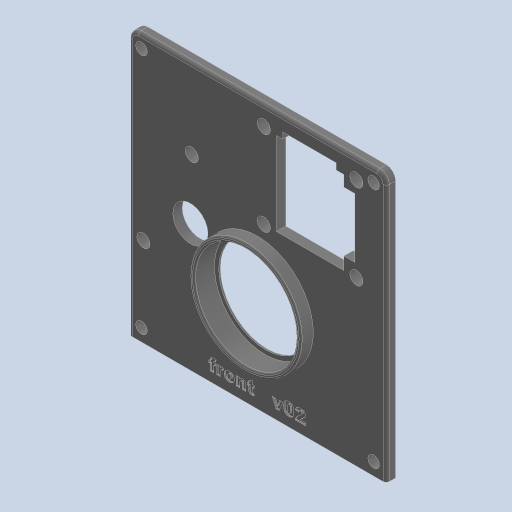
# Autodesk Inventor part: door_front_02
Saved by Autodesk Inventor 2024.4 (Build 284460030, 460C)
## iProperties
Created: 2026-07-13
Part Number: door_front_02
Material: Generic
Document SubType Name: Modeling
Designer: tooles01
Density: 1 g/cm^3
Appearance: Gray
d0: 3.000 mm
d1: 0.00 deg
d3: 32.500 mm
d4: 35.500 mm
d5: 7.000 mm
d6: 0.00 deg
d11: 29.750 mm
d12: 0.500 mm
d13: 0.00 deg
d14: 3.700 mm
d0_1: 36.000 mm
d3_1: 4.900 mm
d4_1: 3.000 mm
d5_1: 10.000 mm
d6_1: 2.000 mm
d7: 2.000 mm
d21: 30.000 mm
d22: 82.000 mm
d23: 4.000 mm
d24: 4.000 mm
d25: 4.000 mm
d26: 4.200 mm
d27: 35.000 mm
d28: 3.000 mm
d29: 4.900 mm
d32: 6.500 mm
d33: 2.000 mm
d34: 2.000 mm
d35: 10.000 mm
d37: 36.000 mm
d38: 2.000 mm
d39: 4.900 mm
d41: 4.200 mm
d48: 1.000 ul
d52: 0.00 deg
d53: 3.000 mm
d54: 34.500 mm
d55: 32.000 mm
d56: 3.000 mm
d57: 2.500 mm
d58: 27.000 mm
d59: 19.000 mm
d60: 7.000 mm
d61: 4.200 mm
d68: 55.000 mm
d69: 3.000 mm
d70: 1.000 mm
d71: 0.500 mm
d72: 40.000 mm
d73: 0.500 mm
d75: 5.000 mm
door_diameter: 36.000 mm
axle_width: 4.900 mm
axle_height: 3.200 mm
handle_height: 10.000 mm
spacing_height: 2.000 mm
spacing_width: 2.000 mm
door_diameter_1: 36.000 mm
handle_height_1: 10.000 mm
spacing_width_1: 2.000 mm
door_spacing_width_1: 2.000 mm
door_handle_height_1: 10.000 mm
door_door_diameter_1: 36.000 mm
door_axle_width_1: 4.900 mm
door_spacing_height_1: 2.000 mm
door_axle_width_2: 4.900 mm
door_axle_height_1: 3.200 mm
door_spacing_height_2: 2.000 mm
d76: 4.000 mm
d77: 9.200 mm
d78: 1.000 mm
d81: 1.000 mm
d83: 17.000 mm
d84: 2.000 mm
d85: 29.500 mm
d86: 6.000 mm
d88: 27.000 mm
d90: 4.000 mm
d91: 4.000 mm
d92: 4.000 mm
d93: 0.500 mm
d94: 1.500 mm
d98: 0.00 deg
d99: 4.000 mm
Author: tooles01
Autodesk Inventor part; units mm, degrees
ref_plane "YZ Plane" through (0, 0, 0) normal (1, 0, 0) x (0, 1, 0)
ref_plane "XZ Plane" through (0, 0, 0) normal (0, 1, 0) x (-1, 0, 0)
ref_plane "XY Plane" through (0, 0, 0) normal (0, 0, 1) x (1, 0, 0)
derived "door_02.ipt"
sketch "Sketch1: base" plane through (0, 0, 0) normal (0, 0, 1) x (1, 0, 0)
  line L0 (-41, 85) -> (41, 85)
  line L1 (41, 85) -> (41, 0)
  line L2 (41, 0) -> (-41, 0)
  line L3 (-41, 0) -> (-41, 85)
  circle A0 centre (0, 30) radius 16.25
  line L4 (-37, 81) -> (37, 81) construction
  line L5 (37, 81) -> (37, 4) construction
  line L6 (37, 4) -> (-37, 4) construction
  line L7 (-37, 4) -> (-37, 81) construction
  point P0 (0, 0)
  point P1 (0, 0)
  point P2 (0, 4)
  dimension "d3" = 32.5
  dimension "d21" = 30
  dimension "d22" = 82
  dimension "d23" = 4
  dimension "d24" = 4
  dimension "d25" = 4
  dimension "d68" = 55
  constraints: 16 end point, 6 perpendicular, 5 coincident, 2 horizontal, 2 midpoint, 2 vertical alignment, 1 centre point
  measures "d3" diameter of A0
  measures "d21" distance from line of L2 A0.centre
  measures "d22" distance of L1.end L2.end
  measures "d23" distance between parallel lines of L2 L6
  measures "d24" distance between parallel lines of L3 L7
  measures "d25" distance between parallel lines of L0 L4
  measures "d68" distance from line of L0 A0.centre
sketch "Sketch2: tube cover/stopper" plane through (0, 0, 0) normal (0, 0, 1) x (1, 0, 0)
  circle A0 centre (0, 30) radius 17.75
  circle A1 centre (0, 30) radius 14.875
  circle A2 centre (0, 30) radius 16.25 projected
  point P0 (0, 0)
  dimension "d4" = 35.5
  dimension "d11" = 29.75
  constraints: 3 coincident, 2 centre point
  measures "d4" diameter of A0
  measures "d11" diameter of A1
sketch "Sketch3: motor & door footprint" plane through (0, 0, 0) normal (0, 0, 1) x (1, 0, 0)
  circle A0 centre (-20.9777, 59.7729) radius 2.1 construction
  circle A1 centre (-36.3835, 28.3459) radius 2.1 construction
  line L0 (-20.9777, 59.7729) -> (-36.3835, 28.3459) construction
  line L1 (-18.8924, 41.9897) -> (-21.0492, 37.5899)
  line L2 (-21.0492, 37.5899) -> (-23.9225, 38.9985)
  line L3 (-23.9225, 38.9985) -> (-21.7657, 43.3982)
  line L4 (-21.7657, 43.3982) -> (-18.8924, 41.9897)
  line L5 (-22.8441, 41.1983) -> (-28.6806, 44.0594) construction
  line L6 (-22.6812, 46.0744) -> (-26.5987, 38.0829)
  line L7 (-26.5987, 38.0829) -> (-17.6195, 33.6813)
  line L8 (-13.7021, 41.6728) -> (-22.6812, 46.0744)
  circle A2 centre (0, 30) radius 18
  line L9 (0, 30) -> (-24.64, 42.0787) construction
  circle A3 centre (0, 30) radius 16.25 construction
  circle A4 centre (-19.0235, 64.2159) radius 18 construction
  line L10 (-25.1952, 47.307) -> (-26.1951, 37.3571) construction
  line L11 (-26.1951, 37.3571) -> (-17.3397, 36.4672) construction
  line L12 (-17.3397, 36.4672) -> (-16.3398, 46.417) construction
  line L13 (-18.8098, 41.8411) -> (-23.6852, 42.331) construction
  line L14 (-23.6852, 42.331) -> (-24.0052, 39.1471) construction
  line L15 (-24.0052, 39.1471) -> (-19.1297, 38.6571) construction
  line L16 (-19.1297, 38.6571) -> (-18.8098, 41.8411) construction
  line L17 (-19.0235, 64.2159) -> (-21.7674, 36.9121) construction
  circle A5 centre (-21.4075, 40.4941) radius 2.45 construction
  point P0 (0, 0)
  point P1 (-19.9708, 39.7898)
  point P2 (-21.5675, 38.9021)
  point P3 (-22.4859, 38.2942)
  point P4 (-18.9698, 40.2491)
  dimension "d26" = 4.2
  dimension "d27" = 34.9999
  dimension "door_axle_height_1" = 3.2
  dimension "door_axle_width_1" = 4.9
  dimension "d32" = 6.5
  dimension "door_spacing_height_1" = 2
  dimension "door_spacing_width_1" = 2
  dimension "door_handle_height_1" = 10
  dimension "door_door_diameter_1" = 36
  dimension "door_spacing_height_2" = 2
  dimension "door_axle_width_2" = 4.9
  constraints: 36 end point, 8 midpoint, 8 perpendicular, 7 parallel, 6 point on circle, 5 centre point, 5 coincident, 4 equal length, 4 point on line, 2 equal radius, 1 collinear, 1 other
  measures "d26" diameter of A0
  measures "d27" distance of L0.start L0.end
  measures "door_axle_height_1" distance of L3.end L1.start
  measures "door_axle_width_1" distance of L1.start L1.end
  measures "d32" distance from line of A0.centre L3
  measures "door_spacing_height_1" distance between parallel lines of L6 L3
  measures "door_spacing_width_1" distance between parallel lines of L8 L4
  measures "door_handle_height_1" distance of L8.start L6.start
  measures "door_door_diameter_1" diameter of A2
  measures "door_spacing_height_2" distance between parallel lines of L11 L15
  measures "door_axle_width_2" diameter of A5
sketch "Sketch4: holes for motor mount" plane through (0, 0, 0) normal (0, 0, 1) x (1, 0, 0)
  circle A0 centre (-21.4075, 40.4941) radius 2.45 construction
  circle A1 centre (-21.4075, 40.4941) radius 5.6
  circle A2 centre (-21.4075, 40.4941) radius 4.6 construction
  point P0 (0, 0)
  point P1 (-20.9777, 59.7729)
  point P2 (-36.3835, 28.3459)
  dimension "d77" = 9.2
  dimension "d78" = 1
  constraints: 2 centre point, 2 coincident
  measures "d77" diameter of A2
  measures "d78" radial gap between concentric circles of A1 A2
sketch "Sketch6: text" plane through (0, 0, 0) normal (0, 0, 1) x (1, 0, 0)
  line L0 (-20, 7) -> (20, 7) construction
  line L1 (20, 7) -> (20, 3) construction
  line L2 (20, 3) -> (-20, 3) construction
  line L3 (-20, 3) -> (-20, 7) construction
  line L4 (-13.9634, 5.8989) -> (-13.4321, 5.8989)
  line L5 (-13.4321, 5.8989) -> (-13.4321, 5.0866)
  line L6 (-13.4321, 5.0866) -> (-13.9634, 5.0866)
  line L7 (-13.9634, 5.0866) -> (-13.9634, 3)
  line L8 (-13.9634, 3) -> (-15.076, 3)
  line L9 (-15.076, 3) -> (-15.076, 5.0866)
  line L10 (-15.076, 5.0866) -> (-15.4918, 5.0866)
  line L11 (-15.4918, 5.0866) -> (-15.4918, 5.8989)
  line L12 (-15.4918, 5.8989) -> (-15.076, 5.8989)
  line L13 (-15.076, 5.8989) -> (-15.076, 6.0298)
  spline S0 degree 2 poles (-15.076, 6.0298) (-15.076, 6.2069) (-14.999, 6.6343) (-14.7911, 6.9038) (-14.41, 7.0693) (-14.0443, 7.0693) knots 0 0 0 1 2 3 4 4 4
  spline S1 degree 2 poles (-14.0443, 7.0693) (-13.7517, 7.0693) (-13.1973, 7) knots 0 0 0 1 1 1
  line L14 (-13.1973, 7) -> (-13.3205, 6.3301)
  spline S2 degree 2 poles (-13.3205, 6.3301) (-13.5168, 6.3609) (-13.64, 6.3609) knots 0 0 0 1 1 1
  spline S3 degree 2 poles (-13.64, 6.3609) (-13.7902, 6.3609) (-13.9211, 6.2608) (-13.948, 6.153) knots 0 0 0 1 2 2 2
  spline S4 degree 2 poles (-13.948, 6.153) (-13.9634, 6.0914) (-13.9634, 5.8989) knots 0 0 0 1 1 1
  line L15 (-13.0125, 5.8989) -> (-11.9731, 5.8989)
  line L16 (-11.9731, 5.8989) -> (-11.9731, 5.4254)
  spline S5 degree 2 poles (-11.9731, 5.4254) (-11.8229, 5.7334) (-11.5034, 5.9644) (-11.2685, 5.9644) knots 0 0 0 1 2 2 2
  spline S6 degree 2 poles (-11.2685, 5.9644) (-11.0221, 5.9644) (-10.7295, 5.8104) knots 0 0 0 1 1 1
  line L17 (-10.7295, 5.8104) -> (-11.0722, 5.0212)
  spline S7 degree 2 poles (-11.0722, 5.0212) (-11.2685, 5.102) (-11.384, 5.102) knots 0 0 0 1 1 1
  spline S8 degree 2 poles (-11.384, 5.102) (-11.6035, 5.102) (-11.7228, 4.9211) knots 0 0 0 1 1 1
  spline S9 degree 2 poles (-11.7228, 4.9211) (-11.8961, 4.667) (-11.8961, 3.9702) knots 0 0 0 1 1 1
  line L18 (-11.8961, 3.9702) -> (-11.8961, 3)
  line L19 (-11.8961, 3) -> (-13.0125, 3)
  line L20 (-13.0125, 3) -> (-13.0125, 5.8989)
  spline S10 degree 2 poles (-10.6756, 4.4398) (-10.6756, 5.1059) (-9.7825, 5.9644) (-9.0202, 5.9644) knots 0 0 0 1 2 2 2
  spline S11 degree 2 poles (-9.0202, 5.9644) (-8.1501, 5.9644) (-7.7074, 5.4601) knots 0 0 0 1 1 1
  spline S12 degree 2 poles (-7.7074, 5.4601) (-7.3494, 5.052) (-7.3494, 4.4591) knots 0 0 0 1 1 1
  spline S13 degree 2 poles (-7.3494, 4.4591) (-7.3494, 3.7892) (-8.2348, 2.9346) (-9.0164, 2.9346) knots 0 0 0 1 2 2 2
  spline S14 degree 2 poles (-9.0164, 2.9346) (-9.717, 2.9346) (-10.1482, 3.2887) knots 0 0 0 1 1 1
  spline S15 degree 2 poles (-10.1482, 3.2887) (-10.6756, 3.7276) (-10.6756, 4.4398) knots 0 0 0 1 1 1
  spline S16 degree 2 poles (-9.563, 4.4437) (-9.563, 4.0549) (-9.2512, 3.6853) (-9.0125, 3.6853) knots 0 0 0 1 2 2 2
  spline S17 degree 2 poles (-9.0125, 3.6853) (-8.7738, 3.6853) (-8.4658, 4.051) (-8.4658, 4.4552) knots 0 0 0 1 2 2 2
  spline S18 degree 2 poles (-8.4658, 4.4552) (-8.4658, 4.8287) (-8.7777, 5.1983) (-9.0048, 5.1983) knots 0 0 0 1 2 2 2
  spline S19 degree 2 poles (-9.0048, 5.1983) (-9.2474, 5.1983) (-9.563, 4.8248) (-9.563, 4.4437) knots 0 0 0 1 2 2 2
  line L21 (-6.8104, 5.8989) -> (-5.7748, 5.8989)
  line L22 (-5.7748, 5.8989) -> (-5.7748, 5.4254)
  spline S20 degree 2 poles (-5.7748, 5.4254) (-5.5438, 5.718) (-5.0664, 5.9644) (-4.7276, 5.9644) knots 0 0 0 1 2 2 2
  spline S21 degree 2 poles (-4.7276, 5.9644) (-4.2656, 5.9644) (-3.7459, 5.4139) (-3.7459, 4.8441) knots 0 0 0 1 2 2 2
  line L23 (-3.7459, 4.8441) -> (-3.7459, 3)
  line L24 (-3.7459, 3) -> (-4.8624, 3)
  line L25 (-4.8624, 3) -> (-4.8624, 4.5938)
  spline S22 degree 2 poles (-4.8624, 4.5938) (-4.8624, 4.8672) (-5.0626, 5.0943) (-5.2474, 5.0943) knots 0 0 0 1 2 2 2
  spline S23 degree 2 poles (-5.2474, 5.0943) (-5.4475, 5.0943) (-5.6978, 4.7902) (-5.6978, 4.3936) knots 0 0 0 1 2 2 2
  line L26 (-5.6978, 4.3936) -> (-5.6978, 3)
  line L27 (-5.6978, 3) -> (-6.8104, 3)
  line L28 (-6.8104, 3) -> (-6.8104, 5.8989)
  line L29 (-1.7401, 7) -> (-1.7401, 5.8989)
  line L30 (-1.7401, 5.8989) -> (-1.128, 5.8989)
  line L31 (-1.128, 5.8989) -> (-1.128, 5.0866)
  line L32 (-1.128, 5.0866) -> (-1.7401, 5.0866)
  line L33 (-1.7401, 5.0866) -> (-1.7401, 4.0587)
  spline S24 degree 2 poles (-1.7401, 4.0587) (-1.7401, 3.8739) (-1.7055, 3.8123) knots 0 0 0 1 1 1
  spline S25 degree 2 poles (-1.7055, 3.8123) (-1.6516, 3.7199) (-1.513, 3.7199) knots 0 0 0 1 1 1
  spline S26 degree 2 poles (-1.513, 3.7199) (-1.3898, 3.7199) (-1.1704, 3.7892) knots 0 0 0 1 1 1
  line L34 (-1.1704, 3.7892) -> (-1.0895, 3.0231)
  spline S27 degree 2 poles (-1.0895, 3.0231) (-1.5014, 2.9346) (-1.8595, 2.9346) knots 0 0 0 1 1 1
  spline S28 degree 2 poles (-1.8595, 2.9346) (-2.2714, 2.9346) (-2.6641, 3.1463) (-2.8527, 3.5813) (-2.8527, 4.0664) knots 0 0 0 1 2 3 3 3
  line L35 (-2.8527, 4.0664) -> (-2.8527, 5.0866)
  line L36 (-2.8527, 5.0866) -> (-3.2608, 5.0866)
  line L37 (-3.2608, 5.0866) -> (-3.2608, 5.8989)
  line L38 (-3.2608, 5.8989) -> (-2.8527, 5.8989)
  line L39 (-2.8527, 5.8989) -> (-2.8527, 6.4302)
  line L40 (-2.8527, 6.4302) -> (-1.7401, 7)
  line L41 (4.666, 5.8989) -> (5.821, 5.8989)
  line L42 (5.821, 5.8989) -> (6.3869, 4.0626)
  line L43 (6.3869, 4.0626) -> (6.9682, 5.8989)
  line L44 (6.9682, 5.8989) -> (8.0885, 5.8989)
  line L45 (8.0885, 5.8989) -> (6.8566, 3)
  line L46 (6.8566, 3) -> (5.871, 3)
  line L47 (5.871, 3) -> (4.666, 5.8989)
  spline S29 degree 2 poles (8.3041, 5.0173) (8.3041, 6.1569) (9.1242, 7.0693) (9.9634, 7.0693) knots 0 0 0 1 2 2 2
  spline S30 degree 2 poles (9.9634, 7.0693) (10.3677, 7.0693) (10.8835, 6.8691) (11.2108, 6.5496) (11.3994, 6.1992) (11.4572, 5.9644) knots 0 0 0 1 2 3 4 4 4
  spline S31 degree 2 poles (11.4572, 5.9644) (11.5688, 5.5178) (11.5688, 5.0289) knots 0 0 0 1 1 1
  spline S32 degree 2 poles (11.5688, 5.0289) (11.5688, 3.9394) (10.8335, 2.9307) (9.9326, 2.9307) knots 0 0 0 1 2 2 2
  spline S33 degree 2 poles (9.9326, 2.9307) (9.4283, 2.9307) (8.8085, 3.2541) (8.6083, 3.5659) knots 0 0 0 1 2 2 2
  spline S34 degree 2 poles (8.6083, 3.5659) (8.4658, 3.7854) (8.3041, 4.5515) (8.3041, 5.0173) knots 0 0 0 1 2 2 2
  spline S35 degree 2 poles (9.4052, 5.0135) (9.4052, 4.2474) (9.6747, 3.6891) (9.9288, 3.6891) knots 0 0 0 1 2 2 2
  spline S36 degree 2 poles (9.9288, 3.6891) (10.0982, 3.6891) (10.3484, 3.9278) (10.4639, 4.4398) (10.4639, 4.9827) knots 0 0 0 1 2 3 3 3
  spline S37 degree 2 poles (10.4639, 4.9827) (10.4639, 5.7796) (10.1944, 6.3301) (9.9249, 6.3301) knots 0 0 0 1 2 2 2
  spline S38 degree 2 poles (9.9249, 6.3301) (9.6516, 6.3301) (9.4052, 5.7719) (9.4052, 5.0135) knots 0 0 0 1 2 2 2
  line L48 (15.2839, 3) -> (11.95, 3)
  spline S39 degree 2 poles (11.95, 3) (12.0077, 3.4928) (12.589, 4.3628) (13.3898, 4.9557) knots 0 0 0 1 2 2 2
  spline S40 degree 2 poles (13.3898, 4.9557) (13.8749, 5.3176) (14.1482, 5.6949) (14.1482, 5.8643) knots 0 0 0 1 2 2 2
  spline S41 degree 2 poles (14.1482, 5.8643) (14.1482, 6.0491) (13.8787, 6.307) (13.6747, 6.307) knots 0 0 0 1 2 2 2
  spline S42 degree 2 poles (13.6747, 6.307) (13.4591, 6.307) (13.1896, 6.0414) (13.1434, 5.7026) knots 0 0 0 1 2 2 2
  line L49 (13.1434, 5.7026) -> (12.0308, 5.7911)
  spline S43 degree 2 poles (12.0308, 5.7911) (12.0962, 6.2608) (12.4466, 6.7883) (13.0818, 7.0693) (13.6439, 7.0693) knots 0 0 0 1 2 3 3 3
  spline S44 degree 2 poles (13.6439, 7.0693) (14.2291, 7.0693) (14.8835, 6.7998) (15.257, 6.2493) (15.257, 5.9028) knots 0 0 0 1 2 3 3 3
  spline S45 degree 2 poles (15.257, 5.9028) (15.257, 5.5371) (14.8296, 4.871) (14.2637, 4.4706) knots 0 0 0 1 2 2 2
  spline S46 degree 2 poles (14.2637, 4.4706) (13.9288, 4.2397) (13.7016, 4.0549) (13.5476, 3.9047) knots 0 0 0 1 2 2 2
  line L50 (13.5476, 3.9047) -> (15.2839, 3.9047)
  line L51 (15.2839, 3.9047) -> (15.2839, 3)
  point P0 (0, 0)
  point P1 (0, 3)
  point P2 (-20, 5)
  dimension "d72" = 40
  dimension "d75" = 5
  dimension "d76" = 4
  constraints: 2 midpoint, 1 horizontal, 1 vertical alignment, 2 other
  measures "d72" distance of L0.start L0.end
  measures "d75" vertical distance of point (0, 0) point (-20, 5)
  measures "d76" distance of L2.end L0.start
extrude "Ex1: base" add sketch "Sketch1: base" along normal blind 3
extrude "Ex2: tube cover" add sketch "Sketch2: tube cover/stopper" along normal blind 7 contours A0
sketch "Sketch5: PCB footprint" plane through (0, 0, 0) normal (0, 0, 1) x (1, 0, 0)
  line L0 (-0.5, 81) -> (34, 81)
  line L1 (34, 81) -> (34, 49)
  line L2 (34, 49) -> (-0.5, 49)
  line L3 (-0.5, 49) -> (-0.5, 81)
  circle A0 centre (2, 79) radius 1.5
  circle A1 centre (31.5, 79) radius 1.5
  circle A2 centre (2, 52) radius 1.5
  circle A3 centre (31.5, 52) radius 1.5
  line L4 (2, 79) -> (31.5, 79) construction
  line L5 (31.5, 79) -> (31.5, 52) construction
  line L6 (31.5, 52) -> (2, 52) construction
  line L7 (2, 52) -> (2, 79) construction
  circle A4 centre (0, 30) radius 17.75 projected
  line L8 (41, 0) -> (41, 85) projected
  line L9 (27.5, 78.5) -> (6, 78.5)
  line L10 (6, 78.5) -> (6, 52)
  line L11 (6, 52) -> (27.5, 52)
  line L12 (27.5, 52) -> (27.5, 78.5)
  line L13 (25, 80.5) -> (8, 80.5)
  line L14 (8, 80.5) -> (8, 78.5)
  line L15 (25, 78.5) -> (25, 80.5)
  circle A5 centre (2, 79) radius 0.5 construction
  line L16 (31, 75) -> (27.5, 75)
  line L17 (27.5, 56) -> (31, 56)
  line L18 (31, 56) -> (31, 75)
  circle A6 centre (31.5, 79) radius 0.5 construction
  circle A7 centre (31.5, 52) radius 0.5 construction
  circle A8 centre (2, 52) radius 0.5 construction
  point P0 (0, 0)
  point P1 (16.75, 79)
  point P2 (16.75, 81)
  dimension "d53" = 3
  dimension "d54" = 34.5
  dimension "d55" = 32
  dimension "d56" = 3
  dimension "d57" = 2.5
  dimension "d58" = 27
  dimension "d59" = 19
  dimension "d60" = 7
  dimension "d81" = 1
  dimension "d83" = 17
  dimension "d84" = 2
  dimension "d85" = 29.5
  dimension "d86" = 6
  dimension "d88" = 27
  dimension "d90" = 4
  dimension "d91" = 4
  dimension "d92" = 4
  dimension "d93" = 0.5
  dimension "d94" = 1.5
  dimension "d99" = 4
  constraints: 36 end point, 15 perpendicular, 8 centre point, 6 equal radius, 5 coincident, 4 point on line, 3 horizontal, 3 horizontal alignment, 3 vertical alignment, 2 midpoint
  measures "d53" diameter of A0
  measures "d54" distance of L0.start L0.end
  measures "d55" distance of L2.end L0.start
  measures "d56" distance from line of L2 A2.centre
  measures "d57" distance from line of A2.centre L3
  measures "d58" distance of L6.end L4.start
  measures "d59" distance from line of A4.centre L2
  measures "d60" distance between parallel lines of L8 L1
  measures "d81" diameter of A5
  measures "d83" distance of L13.start L13.end
  measures "d84" distance of L13.end L14.end
  measures "d85" distance of A5.centre A6.centre
  measures "d86" distance from line of A5.centre L14
  measures "d88" distance of A6.centre A7.centre
  measures "d90" distance from line of A7.centre L17
  measures "d91" distance from line of A6.centre L16
  measures "d92" distance from line of A7.centre L12
  measures "d93" distance from line of L18 A6.centre
  measures "d94" distance from line of L13 A5.centre
  measures "d99" distance from line of A0.centre L10
extrude "Ex3: tube stopper" add sketch "Sketch2: tube cover/stopper" along normal blind 0.5 contours A2
hole "Hole1: mounting (M3 thru holes)" at (-37, 81, 0) at (37, 81, 0) at (-37, 4, 0) at (37, 4, 0) direction (0, 0, 1) diameter 3.7 end through all
hole "Hole2: motor mount (M3 heat-set)" at (-20.9777, 59.7729, 0) at (-36.3835, 28.3459, 0) direction (0, 0, 1) diameter 4.2 end through all
extrude "Ex4: hole for motor" cut sketch "Sketch4: holes for motor mount" along normal through all both and the other way through all
hole "Hole3: PCB holes (M3 heat-set)" at (31.5, 79, 0) at (2, 79, 0) at (2, 52, 0) at (31.5, 52, 0) direction (0, 0, 1) diameter 4.2 end through all
extrude "Ex: space for PCB back" cut sketch "Sketch5: PCB footprint" along normal through all both and the other way through all contours L12 L11 L10 L9 | L9 L14 L13 L15 | L16 L18 L17 L12
extrude "Ex5: text" cut sketch "Sketch6: text" against normal blind 0.5 from surface at 3
fillet "Fillet1" radius 3 2 edges at (41, 85, 1.5) (-41, 85, 1.5)
fillet "Fillet2" radius 1 5 edges at (40.1213, 84.1213, 3) (0, 85, 3) (-40.1213, 84.1213, 3) (-41, 41, 3) (41, 41, 3)
fillet "Fillet3" radius 0.5 2 edges at (-16.25, 30, 7) (-17.75, 30, 7)
equation "\"d24\" = d23"
equation "\"d25\" = d23"
body "Solid1"
